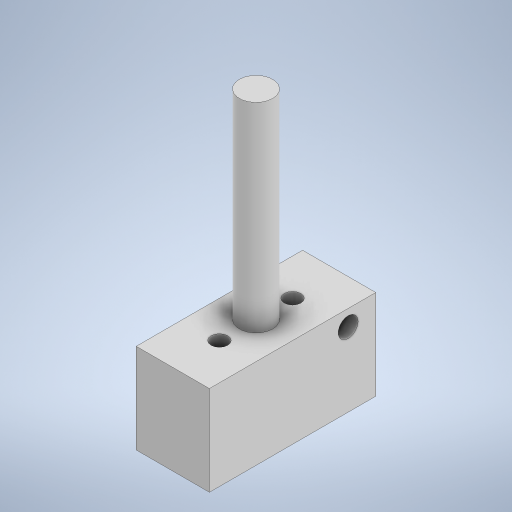
# Autodesk Inventor part: Suporte Eletroimã
Saved by Autodesk Inventor 2023 (Build 270158000, 158)
## iProperties
Created: 2023-03-07
Part Number: Suporte Eletroimã
Material: Genérico
Document SubType Name: Modeling
Designer: Inteli
Density: 1 g/cm^3
Appearance: Padrão
Author: Inteli
Autodesk Inventor part; units mm, degrees
ref_plane "YZ Plane" through (0, 0, 0) normal (1, 0, 0) x (0, 1, 0)
ref_plane "XZ Plane" through (0, 0, 0) normal (0, 1, 0) x (-1, 0, 0)
ref_plane "XY Plane" through (0, 0, 0) normal (0, 0, 1) x (1, 0, 0)
sketch "Esboço1" plane through (0, 0, 0) normal (0, 1, 0) x (-1, 0, 0)
  circle A0 centre (0, 11) radius 10
  circle A1 centre (0, -11) radius 10
  line L0 (9, 2) -> (-9, 2)
  line L1 (-9, -2) -> (9, -2)
  line L2 (9, 20) -> (-9, 20)
  line L3 (-9, -20) -> (9, -20)
  line L4 (11, 25) -> (-11, 25)
  line L5 (-11, 25) -> (-11, -25)
  line L6 (-11, -25) -> (11, -25)
  line L7 (11, -25) -> (11, 25)
  line L8 (9, -20) -> (9, -2)
  line L9 (9, 2) -> (9, 20)
  line L10 (-9, 20) -> (-9, 2)
  line L11 (-9, -2) -> (-9, -20)
  point P0 (-9, 6.6411)
  point P1 (-9, 15.3589)
  point P2 (-4.3589, 20)
  point P3 (4.3589, 20)
  point P4 (9, 15.3589)
  point P5 (9, 6.6411)
  point P6 (4.3589, 2)
  point P7 (-4.3589, 2)
  point P8 (-9, -6.6411)
  point P9 (-4.3589, -2)
  point P10 (4.3589, -2)
  point P11 (9, -6.6411)
  point P12 (9, -15.3589)
  point P13 (4.3589, -20)
  point P14 (-4.3589, -20)
  point P15 (-9, -15.3589)
  point P16 (0, 3)
  point P17 (0, 0)
  dimension "d15" = 22
  dimension "d16" = 40
  dimension "d17" = 18
  dimension "d18" = 22
  dimension "d19" = 50
  constraints: 24 end point, 8 parallel, 3 horizontal, 3 perpendicular, 2 centre point, 1 coincident
  measures "d15" distance of A1.centre point (0, 11)
  measures "d16" distance of L3.start L2.end
  measures "d17" distance of L3.start L3.end
  measures "d18" distance of L6.end L5.end
  measures "d19" distance of L5.end L4.end
extrude "Base Principal dos Imãs" add sketch "Esboço1" along normal blind 18
sketch "Esboço3" plane through (0, 18, 0) normal (0, 1, 0) x (1, 0, 0)
  line L0 (11, -25) -> (11, 25) projected
  line L1 (-11, -25) -> (11, -25)
  line L2 (11, -25) -> (11, 25)
  line L3 (11, 25) -> (-11, 25)
  line L4 (-11, 25) -> (-11, -25)
  line L5 (-11, -25) -> (11, 25) construction
  line L6 (11, -25) -> (-11, 25) construction
  point P0 (0, 0)
  point P1 (11, -25)
  constraints: 12 end point, 2 midpoint, 2 parallel, 1 horizontal, 1 perpendicular
extrude "Extrusão3" add sketch "Esboço3" along normal blind 9
sketch "Esboço4" plane through (0, 27, 0) normal (0, 1, 0) x (1, 0, 0)
  circle A0 centre (0, 0) radius 5
  dimension "d40" = 10
  constraints: 1 centre point, 1 coincident
  measures "d40" diameter of A0
extrude "Extrusão4" add sketch "Esboço4" along normal blind 60
sketch "Esboço5" plane through (-11, 0, -25) normal (-1, 0, 0) x (0, 0, 1)
  line L0 (0.0998, 15) -> (43.9803, 15)
  line L1 (31.6411, 18) -> (40.3589, 18) projected
  circle A0 centre (8.3044, 22.136) radius 3
  line L2 (5, 18) -> (9.6411, 18) projected
  point P0 (25, 0)
  dimension "d43" = 6
  constraints: 1 centre point, 1 horizontal, 3 other
  measures "d43" diameter of A0
extrude "Extrusão5" cut sketch "Esboço5" against normal up to surface (22 mm away)
sketch "Esboço6" plane through (0, 18, 0) normal (0, -1, 0) x (1, 0, 0)
  arc A0 (9, 6.6411) -> (9, 15.3589) centre (0, 11) ccw projected
  arc A1 (9, -15.3589) -> (9, -6.6411) centre (0, -11) ccw projected
  circle A2 centre (0, 11) radius 2.5
  circle A3 centre (0, -11) radius 2.5
  point P0 (0, 0)
  dimension "d48" = 5
  dimension "d49" = 5
  constraints: 4 coincident, 2 centre point
  measures "d48" diameter of A2
  measures "d49" diameter of A3
extrude "Extrusão6" cut sketch "Esboço6" against normal up to surface (9 mm away)
